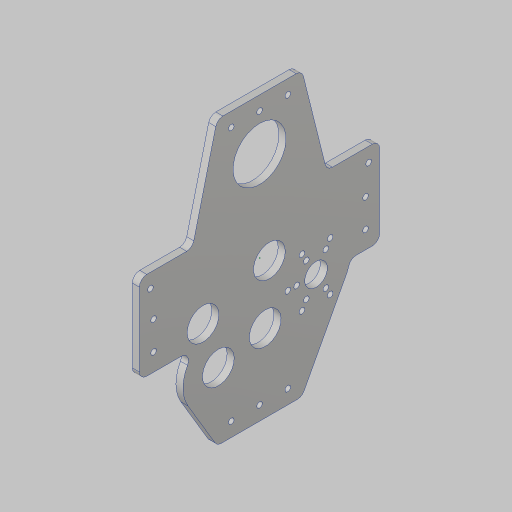
# Autodesk Inventor part: EL2-CGB-001
Saved by Autodesk Inventor 2023.5 (Build 275446000, 446)
## iProperties
Created: 2025-01-19
Part Number: EL2-CGB-001
Material: Aluminum 6061
Document SubType Name: Modeling
Designer: mavericks
Density: 2.7 g/cm^3
Appearance: Aluminum - Flat
Author: mavericks
Autodesk Inventor part; units mm, degrees
ref_plane "YZ Plane" through (0, 0, 0) normal (1, 0, 0) x (0, 1, 0)
ref_plane "XZ Plane" through (0, 0, 0) normal (0, 1, 0) x (-1, 0, 0)
ref_plane "XY Plane" through (0, 0, 0) normal (0, 0, 1) x (1, 0, 0)
sketch "Sketch1" plane through (0, 0, 0) normal (1, 0, 0) x (0, 1, 0)
  line L0 (127, 107.95) -> (-127, 107.95) construction
  line L1 (-127, 107.95) -> (-127, 82.55) construction
  line L2 (-127, 82.55) -> (127, 82.55) construction
  line L3 (127, 82.55) -> (127, 107.95) construction
  line L4 (-44.45, 128.7526) -> (-69.85, 128.7526) construction
  line L5 (-69.85, 128.7526) -> (-69.85, 79.4258) construction
  line L6 (-69.85, 79.4258) -> (-44.45, 79.4258) construction
  line L7 (-44.45, 79.4258) -> (-44.45, 128.7526) construction
  line L8 (69.85, 128.7526) -> (44.45, 128.7526) construction
  line L9 (44.45, 128.7526) -> (44.45, 79.4258) construction
  line L10 (44.45, 79.4258) -> (69.85, 79.4258) construction
  line L11 (69.85, 79.4258) -> (69.85, 128.7526) construction
  line L12 (44.45, 104.0892) -> (-44.45, 104.0892) construction
  line L13 (0, 0) -> (-27.2932, 0) construction
  line L14 (127, -107.95) -> (-127, -107.95) construction
  line L15 (-127, -107.95) -> (-127, -82.55) construction
  line L16 (-127, -82.55) -> (127, -82.55) construction
  line L17 (127, -82.55) -> (127, -107.95) construction
  line L18 (-44.45, -128.7526) -> (-69.85, -128.7526) construction
  line L19 (-69.85, -128.7526) -> (-69.85, -79.4258) construction
  line L20 (-69.85, -79.4258) -> (-44.45, -79.4258) construction
  line L21 (-44.45, -79.4258) -> (-44.45, -128.7526) construction
  line L22 (69.85, -128.7526) -> (44.45, -128.7526) construction
  line L23 (44.45, -128.7526) -> (44.45, -79.4258) construction
  line L24 (44.45, -79.4258) -> (69.85, -79.4258) construction
  line L25 (69.85, -79.4258) -> (69.85, -128.7526) construction
  line L26 (44.45, -104.0892) -> (-44.45, -104.0892) construction
  line L27 (127, 82.55) -> (101.6, 82.55) construction
  line L28 (101.6, 82.55) -> (101.6, -82.55) construction
  line L29 (101.6, -82.55) -> (127, -82.55) construction
  line L30 (127, -82.55) -> (127, 82.55) construction
  line L31 (-127, 82.55) -> (-101.6, 82.55) construction
  line L32 (-101.6, 82.55) -> (-101.6, -82.55) construction
  line L33 (-101.6, -82.55) -> (-127, -82.55) construction
  line L34 (-127, -82.55) -> (-127, 82.55) construction
  point P0 (0, 82.55)
  point P1 (0, 104.0892)
  point P2 (0, -82.55)
  point P3 (0, -104.0892)
  dimension "d0" = 254
  dimension "d1" = 25.4
  dimension "d2" = 82.55
  dimension "d3" = 25.4
  dimension "d4" = 49.3268
  dimension "d6" = 88.9
  dimension "d7" = 3.1242
  dimension "d8" = 25.4
  dimension "d9" = 25.4
  constraints: 70 end point, 16 symmetric about line, 12 parallel, 7 horizontal, 5 perpendicular, 4 midpoint, 2 vertical alignment, 1 horizontal alignment, 1 point on line
  measures "d0" distance of L2.end L1.end
  measures "d1" distance of L1.end L0.end
  measures "d2" vertical distance of L13.start L2.end
  measures "d3" distance of L6.end L5.end
  measures "d4" distance of L5.end L4.end
  measures "d6" distance of L4.start L8.end
  measures "d7" distance from line of L2 L6.end
  measures "d8" distance between parallel lines of L28 L30
  measures "d9" distance between parallel lines of L34 L32
sketch "Sketch2" plane through (0, 0, 0) normal (1, 0, 0) x (0, 1, 0)
  line L0 (-127, 107.95) -> (-127, 82.55) construction
  line L1 (44.45, 104.0892) -> (-44.45, 104.0892) construction
  line L2 (-127, 82.55) -> (127, 82.55) construction
  line L3 (127, 107.95) -> (-127, 107.95) construction
  line L4 (44.45, 79.4258) -> (69.85, 79.4258) construction
  line L5 (127, 82.55) -> (127, 107.95) construction
  line L6 (-69.85, 79.4258) -> (-44.45, 79.4258) construction
  line L7 (-44.45, 79.4258) -> (-44.45, 128.7526) construction
  line L8 (-69.85, 128.7526) -> (-69.85, 79.4258) construction
  line L9 (-44.45, 128.7526) -> (-69.85, 128.7526) construction
  line L10 (101.6, 82.55) -> (101.6, -82.55) construction
  line L11 (127, -82.55) -> (127, 82.55) construction
  line L12 (-127, -82.55) -> (127, -82.55) construction
  line L13 (127, -107.95) -> (-127, -107.95) construction
  line L14 (44.45, -104.0892) -> (-44.45, -104.0892) construction
  line L15 (-127, 82.55) -> (-101.6, 82.55) construction
  line L16 (-101.6, 82.55) -> (-101.6, -82.55) construction
  line L17 (-127, -82.55) -> (-127, 82.55) construction
  line L18 (-69.85, -79.4258) -> (-44.45, -79.4258) construction
  line L19 (-101.6, -82.55) -> (-127, -82.55) construction
  line L20 (-44.45, -79.4258) -> (-44.45, -128.7526) construction
  line L21 (-44.45, -128.7526) -> (-69.85, -128.7526) construction
  line L22 (-69.85, -128.7526) -> (-69.85, -79.4258) construction
  line L23 (-127, -107.95) -> (-127, -82.55) construction
  line L24 (44.45, -79.4258) -> (69.85, -79.4258) construction
  line L25 (44.45, -128.7526) -> (44.45, -79.4258) construction
  line L26 (101.6, -82.55) -> (127, -82.55) construction
  line L27 (69.85, -128.7526) -> (44.45, -128.7526) construction
  line L28 (69.85, -79.4258) -> (69.85, -128.7526) construction
  line L29 (127, -82.55) -> (127, -107.95) construction
  line L30 (69.85, 128.7526) -> (44.45, 128.7526) construction
  line L31 (44.45, 128.7526) -> (44.45, 79.4258) construction
  line L32 (69.85, 79.4258) -> (69.85, 128.7526) construction
  line L33 (127, 82.55) -> (101.6, 82.55) construction
  circle A0 centre (-38.1, -50.8) radius 7.62 construction
  circle A1 centre (-57.15, -5.08) radius 41.91 construction
  circle A2 centre (-57.15, -5.08) radius 11.43 construction
  circle A3 centre (-66.675, 37.0363) radius 31.75 construction
  circle A4 centre (-66.675, 37.0363) radius 15.24 construction
  circle A5 centre (-25.7473, 50.8) radius 27.94 construction
  circle A6 centre (-38.1, -50.8) radius 30.48 construction
  circle A7 centre (-38.1, -50.8) radius 10.16
  circle A8 centre (-57.15, -5.08) radius 14.2875
  circle A9 centre (-66.675, 37.0363) radius 14.2875
  circle A10 centre (-25.7473, 50.8) radius 14.2875
  circle A11 centre (-25.7473, 50.8) radius 20.6375 construction
  circle A12 centre (-66.675, 37.0363) radius 20.6375 construction
  circle A13 centre (-57.15, -5.08) radius 20.6375 construction
  circle A14 centre (-38.1, -50.8) radius 17.4625 construction
  circle A15 centre (-38.1, -50.8) radius 25.4 construction
  line L34 (-41.275, -131.9276) -> (-41.275, -76.2508) construction
  line L35 (-41.275, -76.2508) -> (-73.025, -76.2508) construction
  line L36 (-73.025, -76.2508) -> (-73.025, -131.9276) construction
  line L37 (-73.025, -131.9276) -> (-41.275, -131.9276) construction
  line L38 (-52.3959, -77.7195) -> (-127, -38.1)
  line L39 (-127, -38.1) -> (-127, 38.1)
  line L40 (-127, 38.1) -> (-41.275, 38.1) construction
  line L41 (-41.275, 38.1) -> (-41.275, 104.0892) construction
  arc A16 (-52.3959, -77.7195) -> (-41.275, -81.1142) centre (-38.1, -50.8) ccw
  circle A17 centre (80.9686, 0) radius 23.8125
  circle A18 centre (80.9686, 0) radius 33.3375 construction
  line L42 (37.9487, 60.325) -> (127, 38.1)
  line L43 (127, 38.1) -> (127, -38.1)
  line L44 (127, -38.1) -> (37.9487, -60.325)
  line L45 (37.9487, -60.325) -> (37.9487, -107.95)
  line L46 (37.9487, -107.95) -> (-41.275, -107.95)
  line L47 (-41.275, -107.95) -> (-41.275, -81.1142)
  line L48 (37.9487, 60.325) -> (37.9487, 107.95)
  line L49 (37.9487, 107.95) -> (-41.275, 107.95)
  arc A19 (-23.3654, 68.8297) -> (-38.2397, 37.5831) centre (-25.7473, 50.8) ccw construction
  arc A20 (43.4827, -39.6598) -> (88.1161, 54.1018) centre (80.9686, 0) ccw construction
  line L50 (-41.275, 107.95) -> (-41.275, 56.0863)
  line L51 (-82.9044, 64.325) -> (-127, 38.1)
  arc A21 (-41.275, 56.0863) -> (-82.9044, 64.325) centre (-66.675, 37.0363) ccw
  line L52 (88.1161, 54.1018) -> (-23.3654, 68.8297) construction
  line L53 (43.4827, -39.6598) -> (-38.2397, 37.5831) construction
  circle A22 centre (80.9686, 0) radius 11.1125 construction
  point P0 (25.2487, 98.0186)
  point P1 (0, 95.25)
  point P2 (25.2487, -98.0186)
  point P3 (0, -95.25)
  point P4 (-25.4, -95.25)
  point P5 (-25.4, 95.25)
  point P6 (127, -95.25)
  point P7 (127, 95.25)
  point P8 (0, -82.55)
  point P9 (-114.3, 25.4)
  point P10 (-114.3, 0)
  point P11 (-114.3, -25.4)
  point P12 (-101.6, 0)
  point P13 (-114.3, 82.55)
  point P14 (-38.1, -25.4)
  point P15 (-38.1, -33.3375)
  point P16 (-60.097, -38.1)
  point P17 (-53.223, -42.0688)
  point P18 (-60.097, -63.5)
  point P19 (-53.223, -59.5312)
  point P20 (-38.1, -76.2)
  point P21 (-38.1, -68.2625)
  point P22 (-16.103, -63.5)
  point P23 (-22.977, -59.5313)
  point P24 (-16.103, -38.1)
  point P25 (-22.977, -42.0688)
  point P26 (44.45, 104.0892)
  point P27 (-127, 0)
  point P28 (-127, 0)
  point P29 (101.6, 0)
  point P30 (114.3, 25.4)
  point P31 (114.3, 0)
  point P32 (114.3, -25.4)
  point P33 (114.3, 82.55)
  point P34 (127, 0)
  point P35 (-41.275, -76.8809)
  dimension "d33" = 34.925
  dimension "d34" = 50.8
  dimension "d10" = 15.24
  dimension "d11" = 83.82
  dimension "d12" = 22.86
  dimension "d13" = 63.5
  dimension "d14" = 30.48
  dimension "d15" = 55.88
  dimension "d16" = 60.96
  dimension "d19" = 63.5
  dimension "d23" = 20.32
  dimension "d24" = 28.575
  dimension "d26" = 25.4
  dimension "d27" = 25.4
  dimension "d28" = 25.4
  dimension "d29" = 25.4
  dimension "d30" = 6.35
  dimension "d31" = 6.35
  dimension "d32" = 6.35
  dimension "d37" = 360
  dimension "d41" = 3.175
  dimension "d42" = 76.2
  dimension "d60" = 101.7513
  dimension "d63" = 31.75
  dimension "d64" = 44.45
  dimension "d66" = 34.925
  dimension "d67" = 31.75
  dimension "d68" = 47.625
  dimension "d70" = 9.525
  dimension "d71" = 47.625
  dimension "d73" = 118.1903
  dimension "d74" = 12.7
  dimension "d75" = 36.3728
  dimension "d76" = 109.1438
  dimension "d78" = 9.9314
  dimension "d79" = 9.9314
  dimension "d133" = 205.5979
  dimension "d134" = 45.7518
  dimension "d135" = 112.4501
  dimension "d141" = 22.225
  constraints: 40 end point, 21 centre point, 18 vertical alignment, 15 coincident, 12 point on circle, 11 horizontal alignment, 11 midpoint, 11 point on line, 9 tangent, 3 collinear, 2 equal radius, 2 perpendicular, 1 horizontal, 1 vertical, 20 other
  measures "d10" diameter of A0
  measures "d11" diameter of A1
  measures "d12" diameter of A2
  measures "d13" diameter of A3
  measures "d14" diameter of A4
  measures "d15" diameter of A5
  measures "d16" diameter of A6
  measures "d19" distance from line of L16 A0.centre
  measures "d23" diameter of A7
  measures "d24" diameter of A8
  measures "d26" distance of point (-25.4, 95.25) point (0, 95.25)
  measures "d27" distance of point (25.249, 98.019) point (0, 95.25)
  measures "d28" distance of point (-114.3, 0) point (-114.3, 25.4)
  measures "d29" distance of point (-114.3, 0) point (-114.3, -25.4)
  measures "d30" radial gap between concentric circles of A10 A11
  measures "d31" radial gap between concentric circles of A9 A12
  measures "d32" radial gap between concentric circles of A8 A13
  measures "d41" distance between parallel lines of L20 L34
  measures "d42" distance of L38.end L39.end
  measures "d60" distance from line of L5 point (25.249, 98.019)
  measures "d63" distance from line of L12 A0.centre
  measures "d64" distance from line of L16 A1.centre
  measures "d66" distance from line of L16 A3.centre
  measures "d67" distance from line of L2 A5.centre
  measures "d68" diameter of A17
  measures "d70" radial gap between concentric circles of A17 A18
  measures "d71" distance of L42.start L48.end
  measures "d73" distance of A17.centre A5.centre
  measures "d74" horizontal distance of point (25.249, 98.019) L48.end
  measures "d75" diameter of A19
  measures "d76" diameter of A20
  measures "d78" distance from line of point (25.249, 98.019) L3
  measures "d79" distance from line of L13 point (25.249, -98.019)
  measures "d135" distance of L52.start L52.end
  measures "d141" diameter of A22
extrude "Extrusion1" add sketch "Sketch2" along normal blind 6.35
hole "Mount Holes" at (0, -101.6, 82.55) at (0, -127, 107.95) at (0, -69.85, 79.4258) at (0, 44.45, -79.4258) at (0, 69.85, -79.4258) at (0, 44.45, -128.7526) at (0, 44.45, 128.7526) at (0, 25.2487, 98.0186) at (0, 0, 95.25) at (0, 25.2487, -98.0186) at (0, 0, -95.25) at (0, -25.4, -95.25) at (0, -25.4, 95.25) at (0, -114.3, 25.4) at (0, -114.3, 0) at (0, -114.3, -25.4) at (0, 114.3, 25.4) at (0, 114.3, 0) at (0, 114.3, -25.4) direction (1, 0, 0) diameter 5.1054 end through all clearance for "Flat Head Machine Screw (82)" size "#10" standard "Ansi Unified Screw Threads"
hole "Motor Mount Holes" at (0, -38.1, -33.3375) at (0, -60.097, -38.1) at (0, -53.223, -42.0688) at (0, -60.097, -63.5) at (0, -53.223, -59.5312) at (0, -16.103, -63.5) at (0, -22.977, -59.5313) at (0, -16.103, -38.1) at (0, -22.977, -42.0688) at (0, -38.1, -25.4) direction (1, 0, 0) diameter 5.1054 end through all clearance for "Flat Head Machine Screw (82)" size "#10" standard "Ansi Unified Screw Threads"
sketch "Sketch3" plane through (6.35, 0, 0) normal (1, 0, 0) x (0, 0, -1)
  point P0 (0, 0)
fillet "Fillet1" radius 6.604 12 edges at (3.175, -41.275, 107.95) (3.175, -127, 38.1) (3.175, -127, -38.1) (3.175, -41.275, -81.1142) (3.175, -41.275, -107.95) (3.175, 37.9487, -107.95) (3.175, 37.9487, -60.325) (3.175, 127, -38.1) (3.175, 127, 38.1) (3.175, 37.9487, 60.325) (3.175, 37.9487, 107.95) (3.175, -41.275, 56.0863)
sketch "Sketch7" plane through (6.35, 0, 0) normal (1, 0, 0) x (0, 0, -1)
  arc A0 (-107.95, -34.671) -> (-101.346, -41.275) centre (-101.346, -34.671) ccw construction
  line L0 (-107.95, -34.671) -> (-107.95, 31.3447) construction
  arc A1 (-101.346, 37.9487) -> (-107.95, 31.3447) centre (-101.346, 31.3447) ccw construction
  line L1 (-101.346, 37.9487) -> (-65.4834, 37.9487) construction
  arc A2 (-65.4834, 37.9487) -> (-59.0759, 42.9535) centre (-65.4834, 44.5527) ccw construction
  line L2 (-59.0759, 42.9535) -> (-39.3491, 121.9951) construction
  arc A3 (-32.9416, 127) -> (-39.3491, 121.9951) centre (-32.9416, 120.396) ccw construction
  line L3 (-32.9416, 127) -> (32.9416, 127) construction
  arc A4 (39.3491, 121.9951) -> (32.9416, 127) centre (32.9416, 120.396) ccw construction
  line L4 (39.3491, 121.9951) -> (59.0759, 42.9535) construction
  arc A5 (59.0759, 42.9535) -> (65.4834, 37.9487) centre (65.4834, 44.5527) ccw construction
  line L5 (65.4834, 37.9487) -> (101.346, 37.9487) construction
  arc A6 (107.95, 31.3447) -> (101.346, 37.9487) centre (101.346, 31.3447) ccw construction
  line L6 (107.95, 31.3447) -> (107.95, -34.671) construction
  arc A7 (101.346, -41.275) -> (107.95, -34.671) centre (101.346, -34.671) ccw construction
  line L7 (101.346, -41.275) -> (86.5714, -41.275) construction
  arc A8 (86.5714, -41.275) -> (80.2012, -46.1375) centre (86.5714, -47.879) ccw construction
  arc A9 (77.7195, -52.3959) -> (80.2012, -46.1375) centre (50.8, -38.1) ccw construction
  line L8 (77.7195, -52.3959) -> (39.9622, -123.4934) construction
  arc A10 (34.1297, -127) -> (39.9622, -123.4934) centre (34.1297, -120.396) ccw construction
  line L9 (34.1297, -127) -> (-34.3439, -127) construction
  arc A11 (-40.02, -123.7717) -> (-34.3439, -127) centre (-34.3439, -120.396) ccw construction
  line L10 (-40.02, -123.7717) -> (-64.325, -82.9044) construction
  arc A12 (-64.7124, -51.1154) -> (-64.325, -82.9044) centre (-37.0363, -66.675) ccw construction
  arc A13 (-64.7124, -51.1154) -> (-70.469, -41.275) centre (-70.469, -47.879) ccw construction
  line L11 (-70.469, -41.275) -> (-101.346, -41.275) construction
  circle A14 centre (42.0688, -22.977) radius 2.5527 construction
  circle A15 centre (59.5313, -22.977) radius 2.5527 construction
  circle A16 centre (59.5312, -53.223) radius 2.5527 construction
  circle A17 centre (42.0688, -53.223) radius 2.5527 construction
  circle A18 centre (33.3375, -38.1) radius 2.5527 construction
  circle A19 centre (38.1, -60.097) radius 2.5527 construction
  circle A20 centre (63.5, -60.097) radius 2.5527 construction
  circle A21 centre (63.5, -16.103) radius 2.5527 construction
  circle A22 centre (38.1, -16.103) radius 2.5527 construction
  circle A23 centre (25.4, -38.1) radius 2.5527 construction
  circle A24 centre (0, 114.3) radius 2.5527 construction
  circle A25 centre (25.4, -114.3) radius 2.5527 construction
  circle A26 centre (-25.4, -114.3) radius 2.5527 construction
  circle A27 centre (95.25, -25.4) radius 2.5527 construction
  circle A28 centre (98.0186, 25.2487) radius 2.5527 construction
  circle A29 centre (-98.0186, 25.2487) radius 2.5527 construction
  circle A30 centre (-95.25, 0) radius 2.5527 construction
  circle A31 centre (95.25, 0) radius 2.5527 construction
  circle A32 centre (-95.25, -25.4) radius 2.5527 construction
  circle A33 centre (0, -114.3) radius 2.5527 construction
  circle A34 centre (-25.4, 114.3) radius 2.5527 construction
  circle A35 centre (25.4, 114.3) radius 2.5527 construction
  circle A36 centre (0, 80.9686) radius 23.8125 construction
  circle A37 centre (-50.8, -25.7473) radius 14.2875 construction
  circle A38 centre (-37.0363, -66.675) radius 14.2875 construction
  circle A39 centre (5.08, -57.15) radius 14.2875 construction
  circle A40 centre (50.8, -38.1) radius 10.16 construction
  circle A41 centre (0, 80.9686) radius 54.5719 construction
  circle A42 centre (-50.8, -25.7473) radius 18.1864 construction
  line L12 (-37.5831, -38.2397) -> (39.6598, 43.4827) construction
  line L13 (-54.1018, 88.1161) -> (-68.8297, -23.3654) construction
  circle A43 centre (8.8455, -6.35) radius 14.2875
  circle A44 centre (8.8455, -6.35) radius 18.1864 construction
  line L14 (-7.5115, -23.6556) -> (25.2025, 10.9556) construction
  line L15 (-42.198, -33.8779) -> (35.045, 47.8446) construction
  point P0 (0, 0)
  dimension "d142" = 109.1438
  dimension "d143" = 36.3728
  dimension "d144" = 28.575
  dimension "d145" = 36.3728
  dimension "d148" = 47.625
  dimension "d149" = 6.35
  dimension "d150" = 6.35
  dimension "d160" = 133.35
  dimension "d161" = 99.1045
  constraints: 8 end point, 5 tangent, 4 centre point, 4 coincident, 4 point on circle, 2 parallel, 1 midpoint
  measures "d142" diameter of A41
  measures "d143" diameter of A42
  measures "d144" diameter of A43
  measures "d145" diameter of A44
  measures "d148" distance of L14.start L14.end
  measures "d149" distance between parallel lines of L12 L15
  measures "d150" vertical distance of point (0, 0) A43.centre
  measures "d160" distance from line of A43.centre L3
  measures "d161" distance from line of L6 A44.centre
extrude "Extrusion3" cut sketch "Sketch7" against normal blind 6.35
body "Solid1"
